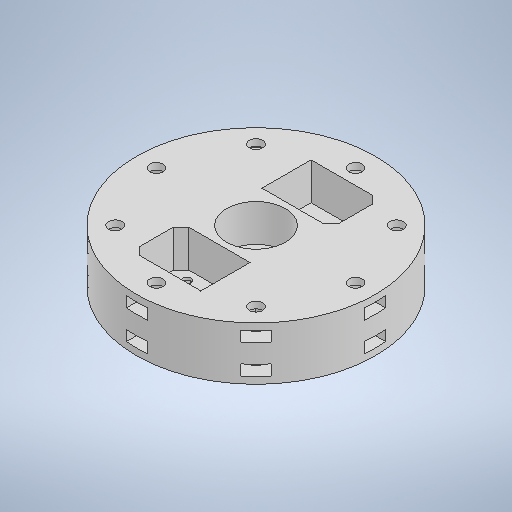
# Autodesk Inventor part: SCARA swivel base - top
Saved by Autodesk Inventor 2025.2 (Build 292293000, 293)
## iProperties
Created: 2025-01-25
Part Number: SCARA swivel base - top
Material: Generic
Document SubType Name: Modeling
Designer: caomi
Density: 1 g/cm^3
Appearance: Default
Author: caomi
Autodesk Inventor part; units mm, degrees
ref_plane "YZ Plane" through (0, 0, 0) normal (1, 0, 0) x (0, 1, 0)
ref_plane "XZ Plane" through (0, 0, 0) normal (0, 1, 0) x (-1, 0, 0)
ref_plane "XY Plane" through (0, 0, 0) normal (0, 0, 1) x (1, 0, 0)
sketch "Sketch1" plane through (0, 0, 0) normal (0, 1, 0) x (-1, 0, 0)
  circle A0 centre (0, 0) radius 45
  line L0 (15, 13.25) -> (-11, 13.25)
  line L1 (-11, 13.25) -> (-11, 31.75)
  line L2 (-11, 31.75) -> (15, 31.75)
  line L3 (45.5655, 22.5) -> (-15.5039, 22.5) construction
  line L4 (0, -63) -> (0, 63) projected
  line L5 (-15, -31.75) -> (11, -31.75)
  line L6 (11, -31.75) -> (11, -13.25)
  line L7 (11, -13.25) -> (-15, -13.25)
  line L8 (19.1191, -22.5) -> (-71.9329, -22.5) construction
  line L9 (69.0652, 0) -> (-95.4326, 0) projected
  circle A1 centre (0, 0) radius 11
  circle A2 centre (0, 0) radius 4
  line L10 (15, 13.25) -> (15, 31.75)
  line L11 (-15, -13.25) -> (-15, -31.75)
  circle A3 centre (9, 28) radius 1.6
  circle A4 centre (-9, -28) radius 1.6
  line L12 (10.7321, 25) -> (7.2679, 25)
  line L13 (7.2679, 25) -> (5.5359, 28)
  line L14 (5.5359, 28) -> (7.2679, 31)
  line L15 (7.2679, 31) -> (10.7321, 31)
  line L16 (10.7321, 31) -> (12.4641, 28)
  line L17 (12.4641, 28) -> (10.7321, 25)
  line L18 (-5.5359, -28) -> (-7.2679, -31)
  line L19 (-7.2679, -31) -> (-10.7321, -31)
  line L20 (-10.7321, -31) -> (-12.4641, -28)
  line L21 (-12.4641, -28) -> (-10.7321, -25)
  line L22 (-10.7321, -25) -> (-7.2679, -25)
  line L23 (-7.2679, -25) -> (-5.5359, -28)
  circle A5 centre (9, 17) radius 1.6
  line L24 (10.7321, 14) -> (7.2679, 14)
  line L25 (7.2679, 14) -> (5.5359, 17)
  line L26 (5.5359, 17) -> (7.2679, 20)
  line L27 (7.2679, 20) -> (10.7321, 20)
  line L28 (10.7321, 20) -> (12.4641, 17)
  line L29 (12.4641, 17) -> (10.7321, 14)
  circle A6 centre (-9, -17) radius 1.6
  line L30 (-5.5359, -17) -> (-7.2679, -20)
  line L31 (-7.2679, -20) -> (-10.7321, -20)
  line L32 (-10.7321, -20) -> (-12.4641, -17)
  line L33 (-12.4641, -17) -> (-10.7321, -14)
  line L34 (-10.7321, -14) -> (-7.2679, -14)
  line L35 (-7.2679, -14) -> (-5.5359, -17)
  point P0 (0, -4.3524)
  point P1 (0, -22.5)
  point P2 (0, 22.5)
  point P3 (0, 22.5)
  point P4 (0, -22.5)
  dimension "d1" = 18.5
  dimension "d2" = 90
  dimension "d12" = 22
  dimension "d26" = 45
  dimension "d50" = 8
  dimension "d53" = 26
  dimension "d54" = 15
  dimension "d55" = 15
  dimension "d56" = 3.2
  dimension "d57" = 6
  dimension "d59" = 6
  dimension "d60" = 6
  dimension "d61" = 6
  dimension "d69" = 3.2
  dimension "d70" = 6
  dimension "d71" = 11
  dimension "d72" = 6
  dimension "d74" = 11
  constraints: 68 end point, 7 centre point, 7 horizontal, 6 coincident, 5 point on line, 5 vertical alignment, 3 perpendicular, 2 parallel, 2 symmetric about line, 2 vertical, 1 equal radius, 1 midpoint, 56 other
  measures "d1" distance of L0.end L1.end
  measures "d2" diameter of A0
  measures "d12" diameter of A1
  measures "d26" distance of point (0, 22.5) point (0, -22.5)
  measures "d50" diameter of A2
  measures "d53" distance of L1.end L2.end
  measures "d54" distance from line of L10 point (0, 22.5)
  measures "d55" distance from line of L11 point (0, -22.5)
  measures "d56" diameter of A3
  measures "d57" distance from line of L10 A3.centre
  measures "d59" distance from line of L11 A4.centre
  measures "d60" distance between parallel lines of L12 L15
  measures "d61" distance between parallel lines of L22 L19
  measures "d69" diameter of A5
  measures "d70" distance between parallel lines of L24 L27
  measures "d71" distance of A5.centre A3.centre
  measures "d72" distance between parallel lines of L34 L31
  measures "d74" distance of A4.centre A6.centre
extrude "Extrusion1" add sketch "Sketch1" along normal blind 20 contours L9 A1 L4 L0 L10 L2 A0 | A0 L4 L5 L6 L7 A1 L9 | L4 L2 L1 L0 A1 L9 A0 | A0 L9 A1 L4 L7 L11 L5 | L4 L0 L1 L2 | L2 L10 L0 L4 | L5 L11 L7 L4 | L4 L7 L6 L5 | A3 | A4 | L12 L13 L14 L15 L16 L17 | L18 L19 L20 L21 L22 L23 | A5 | L24 L25 L26 L27 L28 L29 | A6 | L30 L31 L32 L33 L34 L35
extrude "Extrusion2" cut sketch "Sketch1" against normal blind 14 from surface at 20 contours L4 L0 L1 L2 | L2 L10 L0 L4 | L5 L11 L7 L4 | L4 L7 L6 L5 | A3 | A4 | L12 L13 L14 L15 L16 L17 | L18 L19 L20 L21 L22 L23 | A5 | L24 L25 L26 L27 L28 L29 | A6 | L30 L31 L32 L33 L34 L35
extrude "Extrusion9" cut sketch "Sketch1" along normal blind 5 contours A3 | A4 | L12 L13 L14 L15 L16 L17 | L18 L19 L20 L21 L22 L23 | A5 | L24 L25 L26 L27 L28 L29 | A6 | L30 L31 L32 L33 L34 L35
extrude "Extrusion10" cut sketch "Sketch1" along normal up to surface (6 mm away) contours A3 | A4 | A5 | A6
extrude "Extrusion6" add sketch "Sketch1" along normal up to surface (6 mm away) contours A1 L4 A2 L9 | L9 A2 L4 A1 | A2 L4 L9 | L9 L4 A2 | L4 A2 L9 A1 | A1 L9 A2 L4 | L9 A2 L4 | L4 A2 L9
sketch "Sketch4" plane through (0, 20, 0) normal (0, 1, 0) x (1, 0, 0)
  circle A0 centre (-37.5, 0) radius 2.5
  line L0 (-52.889, 4) -> (-35.4144, 4)
  line L1 (-35.4144, 4) -> (-33.105, 0)
  line L2 (-33.105, 0) -> (-35.4144, -4)
  line L3 (-35.4144, -4) -> (-52.889, -4)
  line L4 (-52.889, -4) -> (-52.889, 4)
  line L5 (0, 0) -> (-69.9236, 0) construction
  circle A1 centre (0, 0) radius 45 projected
  dimension "d32" = 5
  dimension "d33" = 60
  dimension "d34" = 8
  dimension "d35" = 4.395
  dimension "d44" = 37.5
  constraints: 12 end point, 2 horizontal, 1 centre point, 1 parallel, 1 point on line, 1 vertical, 2 other
  measures "d32" diameter of A0
  measures "d33" angle of L1 L5
  measures "d34" distance between parallel lines of L0 L3
  measures "d35" distance of L1.end A0.centre
  measures "d44" distance of A0.centre A1.centre
ref_plane "Work Plane2" through (0, 15.5, 0) normal (0, 1, 0) x (1, 0, 0)
ref_plane "Work Plane3" through (0, 4.5, 0) normal (0, 1, 0) x (1, 0, 0)
extrude "Extrusion4" cut sketch "Sketch4" along normal mid plane 4 from surface at -15.5 contours A0 | L0 A1 L3 L4 | L0 L1 L2 L3 A1 picked at (-39.5409, -3.4458)
extrude "Extrusion5" cut sketch "Sketch4" along normal mid plane 4 from surface at -4.5 contours A0 | L0 A1 L3 L4 | L0 L1 L2 L3 A1 picked at (-39.5409, -3.4458)
extrude "Extrusion7" cut sketch "Sketch4" against normal up to surface (20 mm away) contours A0
pattern_circular "Circular Pattern1" count 8 over 360 about axis through (0, 0, 0) along (0, 1, 0) of "Extrusion5", "Extrusion4", "Extrusion7"
chamfer "Chamfer1" distance 3 angle 45 4 edges at (-15, 13, 31.75) (-15, 13, 13.25) (15, 13, -13.25) (15, 13, -31.75)
body "Solid1"
